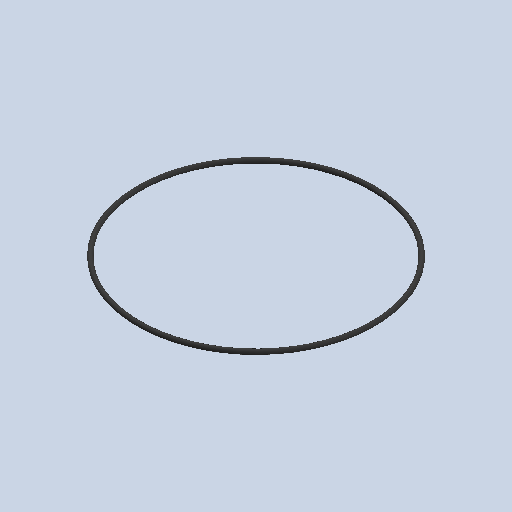
# Autodesk Inventor part: 1.78
Saved by Autodesk Inventor 2025.3 (Build 293356030, 356C)
## iProperties
Created: 2024-12-23
Part Number: 1.78
Material: Caucho
Document SubType Name: Modeling
Designer: Usuario
Density: 0.93 g/cm^3
Appearance: Caucho - Negro
Mass: 0.611083 g
Surface Area: 14.7658 cm^2
Volume: 0.657079 cm^3
Author: Usuario
Autodesk Inventor part; units mm, degrees
ref_plane "YZ Plane" through (0, 0, 0) normal (1, 0, 0) x (0, 1, 0)
ref_plane "XZ Plane" through (0, 0, 0) normal (0, 1, 0) x (-1, 0, 0)
ref_plane "XY Plane" through (0, 0, 0) normal (0, 0, 1) x (1, 0, 0)
sketch "Boceto1" plane through (0, 0, 0) normal (0, 0, 1) x (1, 0, 0)
  circle A0 centre (45.2, 0) radius 0.89
  line L0 (0, -10.2838) -> (0, 10.2838)
  line L1 (0, 0) -> (45.2, 0) construction
  point P0 (44.31, 0)
  dimension "d0" = 1.78
  dimension "d4" = 88.62
  constraints: 4 end point, 1 horizontal, 1 horizontal alignment, 1 midpoint, 1 perpendicular, 1 point on line, 2 other
  measures "d4" diameter of point (44.31, 0) L0
revolve "Revolución1" add sketch "Boceto1" angle 360 about axis through (0, -10.2838, 0) along (0, 1, 0)
sketch "Boceto2" plane through (0, 0, 0) normal (0, 0, 1) x (1, 0, 0)
  line L0 (0, -10.2838) -> (0, 10.2838) projected
  circle A0 centre (37.265, 0) radius 0.89
  point P0 (0, 0)
  point P1 (0, 0)
  point P2 (36.375, 0)
  dimension "d5" = 1.78
  dimension "d6" = 72.75
  constraints: 3 horizontal alignment, 1 midpoint, 2 other
  measures "d6" diameter of point (36.375, 0) L0
revolve "Revolución2" [suppressed]
equation "\"d5\" = d0"
